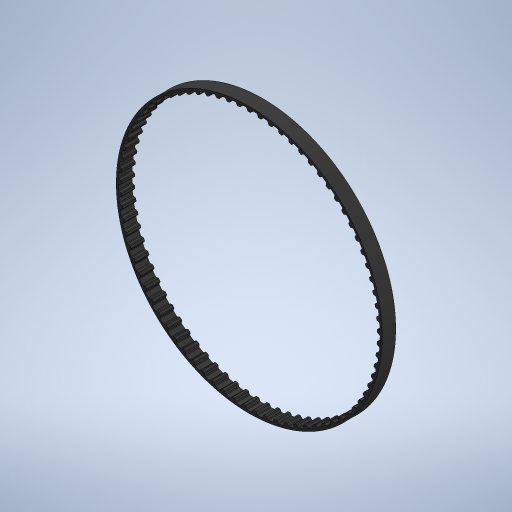
# Autodesk Inventor part: XL Belt Generator
Saved by Autodesk Inventor 2023 (Build 270158000, 158)
## iProperties
RuleStatus: InUse
Created: 2022-06-22
Part Number: XL Belt Generator
Material: Rubber
Document SubType Name: Modeling
Designer: Nathan Cai
Density: 0.93 g/cm^3
Appearance: Rubber - Black
Mass: 3.49489 g
Surface Area: 67.8029 cm^2
Volume: 3.75794 cm^3
Author: Nathan Cai
Autodesk Inventor part; units mm, degrees
ref_plane "YZ Plane" through (0, 0, 0) normal (1, 0, 0) x (0, 1, 0)
ref_plane "XZ Plane" through (0, 0, 0) normal (0, 1, 0) x (-1, 0, 0)
ref_plane "XY Plane" through (0, 0, 0) normal (0, 0, 1) x (1, 0, 0)
sketch "Sketch1" plane through (0, 0, 0) normal (0, 0, 1) x (1, 0, 0)
  circle A0 centre (0, 0) radius 62.255 construction
  line L0 (0, 0) -> (0, 62.255) construction
  line L1 (0, 0) -> (5.0744, 62.0479) construction
  arc A1 (4.9904, 61.0213) -> (0, 61.225) centre (0, 0) ccw construction
  arc A2 (5.0324, 61.5346) -> (0, 61.74) centre (0, 0) ccw construction
  arc A3 (0.4389, 59.9534) -> (0, 59.955) centre (0, 0) ccw
  line L2 (0, 0) -> (0.6941, 61.2211) construction
  line L3 (0.7843, 60.1689) -> (1.1788, 60.9905)
  arc A4 (0.4389, 59.9534) -> (0.7843, 60.1689) centre (0.4417, 60.3334) ccw
  line L4 (0, 0) -> (2.5183, 61.6887) construction
  arc A5 (2.4973, 61.1741) -> (1.5308, 61.2059) centre (0, 0) ccw
  arc A6 (1.5308, 61.2059) -> (1.1788, 60.9905) centre (1.5213, 60.826) ccw
  arc A7 (4.8869, 59.7556) -> (4.4493, 59.7897) centre (0, 0) ccw
  line L5 (4.1227, 60.0327) -> (3.7965, 60.8837)
  arc A8 (4.1227, 60.0327) -> (4.4493, 59.7897) centre (4.4775, 60.1687) ccw
  arc A9 (3.4631, 61.127) -> (2.4973, 61.1741) centre (0, 0) ccw
  arc A10 (3.7965, 60.8837) -> (3.4631, 61.127) centre (3.4416, 60.7476) ccw
  line L6 (1.2849, 61.2116) -> (0, 0) construction
  line L7 (0, 59.955) -> (0, 62.255)
  line L8 (4.8869, 59.7556) -> (5.0744, 62.0479)
  arc A11 (5.0744, 62.0479) -> (0, 62.255) centre (0, 0) ccw
  point P0 (0.6797, 59.9512)
  dimension "PD" = 124.5101
  dimension "pArcDeg" = 4.675
  dimension "standardSpineThickness" = 1.03
  dimension "centerLine" = 0.515
  dimension "toothHeight" = 1.27
  dimension "d7" = 25
  dimension "d8" = 0.38
  dimension "d9" = 0.38
  dimension "toothArcLength" = 1.203
  dimension "innerRadius" = 61.2251
  constraints: 30 point on circle, 18 end point, 12 centre point, 7 point on line, 7 symmetric about line, 5 coincident, 4 tangent, 2 vertical, 1 collinear, 4 other
  measures "PD" diameter of A0
  measures "pArcDeg" angle of L0 L1
  measures "standardSpineThickness" radial gap between concentric circles of A0 A1
  measures "centerLine" radial gap between concentric circles of A0 A2
  measures "toothHeight" radial gap between concentric circles of A1 A3
  measures "d7" angle of L2 L3
  measures "d8" radius of A4
  measures "d9" radius of A6
  measures "toothArcLength" angle of L0 L6
  measures "innerRadius" radius of A1
extrude "Extrusion2" add sketch "Sketch1" along normal blind 6.35
pattern_circular "Circular Pattern1" count 77 over 360 about axis through (0, 0, 0) along (0, 0, 1) of "Extrusion2"
equation "\"centerLine\" = 0.5 * standardSpineThickness"
equation "\"d9\" = d8"
equation "\"p\" = 5.08"
equation "\"w\" = 6.35"
body "Solid2"
